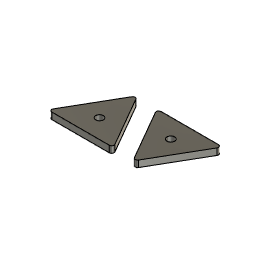
diamondFileHolder_60degrees (Autodesk Fusion 360 design; units mm, degrees)
Autodesk Fusion 360 part; units mm, degrees
sketch "Sketch1" plane through (0, 0, 0) normal (0, 0, 1) x (1, 0, 0) in component "plate"
  line L0 (3.81, 0) -> (78.74, 0)
  line L1 (82.55, 3.81) -> (82.55, 46.99)
  line L2 (78.74, 50.8) -> (3.81, 50.8)
  line L3 (0, 46.99) -> (0, 3.81)
  arc A0 (3.81, 50.8) -> (0, 46.99) centre (3.81, 46.99) ccw
  arc A1 (82.55, 46.99) -> (78.74, 50.8) centre (78.74, 46.99) ccw
  arc A2 (78.74, 0) -> (82.55, 3.81) centre (78.74, 3.81) ccw
  arc A3 (0, 3.81) -> (3.81, 0) centre (3.81, 3.81) ccw
  point P0 (82.55, 0)
  point P1 (0, 50.8)
  dimension "d1" = 82.55
  dimension "d2" = 50.8
  dimension "d3" = 3.81
  constraint horizontal L0
  constraint vertical L1
  constraint horizontal L2
  constraint vertical L3
  constraint coincident P1 L2
  constraint coincident P1 L3
  constraint tangent L2 A0
  constraint tangent L3 A0
  constraint tangent L1 A1
  constraint tangent L2 A1
  constraint equal A0 A1
  constraint coincident P0 L0
  constraint coincident P0 L1
  constraint tangent L0 A2
  constraint tangent L1 A2
  constraint equal A0 A2
  constraint coincident origin L0
  constraint coincident origin L3
  constraint tangent L0 A3
  constraint tangent L3 A3
  constraint equal A0 A3
  measures "d1" distance of origin P0
  measures "d2" distance of origin P1
  measures "d3" radius of A0
extrude "Extrude1" add sketch "Sketch1" along normal blind 1.27 makes body 1 in component "plate"
sketch "Sketch1 (2)" plane through (0, 0, 0) normal (1, 0, 0) x (0, 1, 0) in component "holder"
  line L0 (56.2325, -2.54) -> (-5.4325, -2.54)
  line L1 (-7.6322, 1.27) -> (23.2003, 54.6735)
  line L2 (27.5997, 54.6735) -> (58.4322, 1.27)
  line L3 (46.99, 0) -> (3.81, 0)
  line L4 (50.8, 0) -> (46.99, 0)
  line L5 (3.81, 0) -> (0, 0)
  line L6 (25.4, 0) -> (25.4, -2.54) construction
  line L7 (50.8, 1.27) -> (46.99, 1.27) construction
  line L8 (46.99, 1.27) -> (3.81, 1.27) construction
  line L9 (3.81, 1.27) -> (0, 1.27) construction
  line L10 (50.8, 1.27) -> (0, 1.27) construction
  line L11 (0, 1.27) -> (0, 0) construction
  line L12 (0, 0) -> (50.8, 0) construction
  line L13 (50.8, 0) -> (50.8, 1.27) construction
  line L14 (-0.127, -0.127) -> (50.927, -0.127)
  line L15 (50.927, -0.127) -> (50.927, 1.397) construction
  line L16 (50.927, 1.397) -> (-0.127, 1.397)
  line L17 (-0.127, 1.397) -> (-0.127, -0.127) construction
  arc A0 (27.5997, 54.6735) -> (23.2003, 54.6735) centre (25.4, 53.4035) ccw
  arc A1 (56.2325, -2.54) -> (58.4322, 1.27) centre (56.2325, 0) ccw
  arc A2 (-7.6322, 1.27) -> (-5.4325, -2.54) centre (-5.4325, 0) ccw
  arc A3 (50.927, -0.127) -> (50.927, 1.397) centre (50.927, 0.635) ccw
  arc A4 (-0.127, 1.397) -> (-0.127, -0.127) centre (-0.127, 0.635) ccw
  arc A5 (52.3699, 3.8962) -> (53.6897, 4.6582) centre (53.0298, 4.2772) ccw
  line L18 (53.6897, 4.6582) -> (28.1627, 48.8723)
  line L19 (26.8429, 48.1103) -> (52.3699, 3.8962)
  arc A6 (28.1627, 48.8723) -> (26.8429, 48.1103) centre (27.5028, 48.4913) ccw
  arc A7 (23.9571, 48.1103) -> (22.6373, 48.8723) centre (23.2972, 48.4913) ccw
  line L20 (22.6373, 48.8723) -> (-2.8897, 4.6582)
  line L21 (-1.5699, 3.8962) -> (23.9571, 48.1103)
  arc A8 (-2.8897, 4.6582) -> (-1.5699, 3.8962) centre (-2.2298, 4.2772) ccw
  circle A9 centre (25.4, 17.8012) radius 4.064
  line L22 (43.016, 27.9717) -> (18.9016, 14.0493) construction
  line L23 (7.784, 27.9717) -> (30.3338, 14.9526) construction
  line L24 (25.4, -2.54) -> (25.4, 29.45) construction
  point P0 (25.4, 17.8012)
  dimension "d7" = 2.54
  dimension "d8" = 0.127
  dimension "d11" = 2.54
  dimension "d12" = 2.54
  dimension "d13" = 2.54
  dimension "d15" = 360
  dimension "d16" = 8.128
  constraint horizontal L0
  constraint midpoint L3 L6.start
  constraint perpendicular L0 L6
  constraint coincident L0 L6.end
  constraint horizontal L10
  constraint vertical L11
  constraint horizontal L12
  constraint vertical L13
  constraint coincident L5.end L11.end
  constraint coincident L7.start L10.start
  constraint tangent L2 A0
  constraint tangent L1 A0
  constraint tangent L2 A1
  constraint tangent L0 A1
  constraint tangent L0 A2
  constraint tangent L1 A2
  constraint midpoint L15 A3.centre
  constraint symmetric L6 L14.end L14.start
  constraint symmetric L6 L15.end L16.end
  constraint symmetric L6 A3 A4
  constraint coincident P0 A9.centre
  constraint midpoint L2 L22.start
  constraint perpendicular L2 L22
  constraint midpoint L1 L23.start
  constraint perpendicular L1 L23
  constraint equal L0 L2
  constraint equal L0 L1
  constraint midpoint L0 L6.end
  constraint perpendicular L0 L24
  constraint coincident P0 L23
  constraint coincident P0 L22
  constraint collinear L6 L24
  measures "d7" distance of L6.start L6.end
  measures "d11" radius of A0
  measures "d12" radius of A1
  measures "d13" radius of A2
  measures "d16" diameter of A9
extrude "Extrude1'" add sketch "Sketch1 (2)" along normal blind 7 separate body contours L0 L1 L2 A0 A1 A2 | L14 L16 A3 A4 | A5 L18 L19 A6 | A7 L20 L21 A8 makes body 2 in component "holder"
extrude "Extrude2" cut sketch "Sketch1 (2)" along normal blind 2.54 contours L14 L16 A3 A4 | A5 L18 L19 A6 | A7 L20 L21 A8 bodies 2 in component "holder"
copy_body "CutPasteBodies1" bodies 2 removing the originals makes body 3 in component "holder"
sketch "Sketch1 (3)" plane through (0, 0, 0) normal (0, 0, 1) x (1, 0, 0) in component "mdf"
  line L0 (0, 0) -> (203.2, 0)
  line L1 (203.2, 0) -> (203.2, 88.9)
  line L2 (203.2, 88.9) -> (0, 88.9)
  line L3 (0, 88.9) -> (0, 0)
  dimension "d21" = 203.2
  dimension "d22" = 88.9
  constraint horizontal L0
  constraint vertical L1
  constraint horizontal L2
  constraint vertical L3
  constraint coincident L0.start L3.end
  measures "d21" distance of L0.start L0.end
  measures "d22" distance of L0.start L2.end
extrude "Extrude1''" add sketch "Sketch1 (3)" along normal blind 7 separate body makes body 4 in component "mdf"
component "plate" placed x (1, 0, 0) y (0, 1, 0) z (0, 0, 1) at (-75.184, 0, 0)
component "holder" placed x (1, 0, 0) y (0, 1, 0) z (0, 0, 1) at (0, 0, 0)
component "mdf" placed x (1, 0, 0) y (0, 1, 0) z (0, 0, 1) at (0, 0, 0)
component "holder" placed x (0, 0, 1) y (0.5, 0.866025, 0) z (-0.866025, 0.5, 0) at (134.5, 24.4841, -0.0473)
